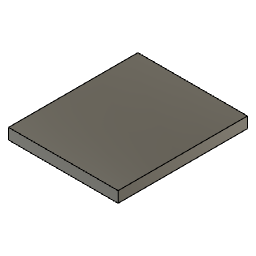
Resistor Pins Floor (Autodesk Fusion 360 design; units mm, degrees)
Autodesk Fusion 360 part; units mm, degrees
sketch "Sketch1" plane through (0, 0, 0) normal (0, 0, 1) x (1, 0, 0)
  line L0 (0, 0) -> (50, 0)
  line L1 (50, 0) -> (50, -59)
  line L2 (50, -59) -> (0, -59)
  line L3 (0, -59) -> (0, 0)
  dimension "d7" = 50
  dimension "d8" = 59
  constraint horizontal L0
  constraint vertical L1
  constraint horizontal L2
  constraint vertical L3
  constraint coincident L0.start L3.end
  measures "d7" distance of L0.start L0.end
  measures "d8" distance of L0.start L2.end
extrude "Extrude1" add sketch "Sketch1" along normal blind 5
equation "perfboard_length = 39 mm"
equation "perfboard_width = 30 mm"
equation "width = perfboard_length + 2 * screw_radius * 2"
equation "length = perfboard_width + 2 * screw_radius * 2"
equation "height = 5 mm"
equation "d7 = length"
equation "d8 = width"
equation "d9 = height"
equation "extra = 100 mm"
equation "screw_radius = 5 mm"
